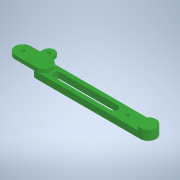
# Autodesk Inventor part: pieza3parte3
Saved by Autodesk Inventor 2021 (Build 250183000, 183)
## iProperties
Created: 2021-03-25
Part Number: pieza3parte3
Material: Genérico
Document SubType Name: Modeling
Designer: Arturo
Density: 1 g/cm^3
Appearance: Suave - Verde bosque oscuro
Author: Arturo
Autodesk Inventor part; units mm, degrees
ref_plane "YZ Plane" through (0, 0, 0) normal (1, 0, 0) x (0, 1, 0)
ref_plane "XZ Plane" through (0, 0, 0) normal (0, 1, 0) x (-1, 0, 0)
ref_plane "XY Plane" through (0, 0, 0) normal (0, 0, 1) x (1, 0, 0)
sketch "Boceto1" plane through (0, 0, 0) normal (0, 1, 0) x (-1, 0, 0)
  circle A0 centre (0, 0) radius 7.5
  circle A1 centre (20, 0) radius 1.75
  arc A2 (87.5, -3.5) -> (87.5, 3.5) centre (87.5, 0) ccw
  arc A3 (32.5, 3.5) -> (32.5, -3.5) centre (32.5, 0) ccw
  line L0 (100, -7.5) -> (0, -7.5)
  line L1 (100, 7.5) -> (0, 7.5)
  line L2 (87.5, -3.5) -> (32.5, -3.5)
  line L3 (87.5, 3.5) -> (32.5, 3.5)
  arc A4 (105, 2.5) -> (100, 7.5) centre (100, 2.5) ccw
  arc A5 (100, -7.5) -> (105, -2.5) centre (100, -2.5) ccw
  line L4 (105, 2.5) -> (105, -2.5)
  dimension "d0" = 15
  dimension "d3" = 3.5
  dimension "d5" = 7
  dimension "d7" = 7
  dimension "d10" = 100
  dimension "d12" = 55
  dimension "d13" = 55
  constraints: 10 end point, 10 point on circle, 6 centre point, 1 coincident, 1 vertical
  measures "d0" diameter of A0
  measures "d3" diameter of A1
  measures "d5" diameter of A2
  measures "d7" diameter of A3
  measures "d10" distance of L0.start L0.end
  measures "d12" distance of L2.start L2.end
  measures "d13" distance of L3.start L3.end
extrude "Extrusión1" add sketch "Boceto1" along normal blind 9 contours A0
extrude "Extrusión2" add sketch "Boceto1" along normal blind 6 contours A0 L1 A4 L4 A5 L0
sketch "Boceto2" plane through (0, 6, 0) normal (0, 1, 0) x (1, 0, 0)
  line L0 (-100, -7.5) -> (0, -7.5) projected
  arc A0 (0, 7.5) -> (0, -7.5) centre (0, 0) ccw projected
  line L1 (0, 7.5) -> (-100, 7.5) projected
  arc A1 (-100, 7.5) -> (-105, 2.5) centre (-100, 2.5) ccw projected
  line L2 (-105, 2.5) -> (-105, -2.5) projected
  arc A2 (-105, -2.5) -> (-100, -7.5) centre (-100, -2.5) ccw projected
  line L3 (-87.5, 3.5) -> (-32.5, 3.5) projected
  arc A3 (-32.5, -3.5) -> (-32.5, 3.5) centre (-32.5, 0) ccw projected
  line L4 (-32.5, -3.5) -> (-87.5, -3.5) projected
  arc A4 (-87.5, 3.5) -> (-87.5, -3.5) centre (-87.5, 0) ccw projected
  circle A5 centre (-20, 0) radius 1.75 projected
  arc A6 (-100, -7.5) -> (-100, 7.5) centre (-100, 0) ccw
  circle A7 centre (-120, 0) radius 1.75
  arc A8 (-120, 7.5) -> (-120, -7.5) centre (-120, 0) ccw
  line L5 (-120, -7.5) -> (-100, -7.5)
  line L6 (-120, 7.5) -> (-100, 7.5)
  dimension "d22" = 15
  dimension "d24" = 3.5
  dimension "d25" = 15
  dimension "d26" = 20
  dimension "d27" = 20
  constraints: 4 end point, 4 point on circle, 3 centre point, 2 tangent, 1 coincident, 1 horizontal
  measures "d22" diameter of A6
  measures "d24" diameter of A7
  measures "d25" diameter of A8
  measures "d26" distance of L5.start L0.start
  measures "d27" distance of L6.start L1.end
extrude "Extrusión3" add sketch "Boceto2" along normal blind 3.5 contours L5 A8 L6 A1 L2 A2 | A2 L2 A1 A6
sketch "Boceto3" plane through (0, 9.5, 0) normal (0, 1, 0) x (1, 0, 0)
  line L0 (-87.5, 3.5) -> (-32.5, 3.5) projected
  line L1 (-120, -7.5) -> (-100, -7.5) projected
  arc A0 (-100, -7.5) -> (-100, 7.5) centre (-100, 0) ccw projected
  line L2 (-100, 7.5) -> (-120, 7.5) projected
  arc A1 (-120, 7.5) -> (-120, -7.5) centre (-120, 0) ccw projected
  circle A2 centre (-120, 0) radius 1.75 projected
  line L3 (0, 7.5) -> (-100, 7.5) projected
  line L4 (-100, 7.5) -> (-100, 10.5)
  circle A3 centre (-105.9988, 10.6207) radius 1.5
  arc A4 (-100, 10.5) -> (-111.9976, 10.5) centre (-105.9988, 10.6207) ccw
  arc A5 (-100, 7.5) -> (-105, 2.5) centre (-100, 2.5) ccw projected
  line L5 (-111, 7.5) -> (-100, 7.5)
  line L6 (-111.9976, 10.5) -> (-111.9976, 7.5)
  point P0 (0, 0)
  dimension "d32" = 3
  dimension "d37" = 6
  dimension "d38" = 3
  dimension "d39" = 3
  constraints: 6 end point, 2 centre point, 2 point on circle, 2 point on line, 2 vertical, 1 coincident, 1 collinear, 1 tangent
  measures "d32" diameter of A3
  measures "d37" radius of A4
  measures "d38" distance of L2.start L4.end
  measures "d39" distance of L6.start L6.end
extrude "Extrusión4" add sketch "Boceto3" against normal blind 2.5 contours L2 L6 A4 L4
